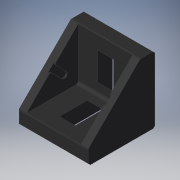
# Autodesk Inventor part: 14073
Saved by Autodesk Inventor 2019 (Build 230136000, 136)
## iProperties
Created: 2023-03-27
Part Number: 14073
Material: Generic
Catalog Web Link: www.cadenas.de
Description: 14071, 14073-2 Hole Inside Corner Brackets
Vendor: 8020
Document SubType Name: Modeling
Designer: psAdmin
Manufacturer: 8020
Mass: 7.49289 g
Surface Area: 51.4239 cm^2
Volume: 7.49289 cm^3
Density: 1 g/cm^3
Appearance: PSOLRGB-175-175-175
Category: PARTsolutions
Company: 8020
Title: 14073
Author: Cadenas PARTsolutions
Comments: 2 Hole Inside Corner Brackets
PSOL_IDENT_0: {$CADENAS_DATA/23d-libs/8020/metric/joining_plates/14071.prj},157 {VTYP=3D},{NB=14073},{LINA=14073},
PSOL_IDENT_1: {NN=14071, 14073},{DATE=31.07.2020 09:21:28},{GEOMDATE=27.02.2012 05:57:00},{VERSION=},{LINEID=10},{
PSOL_IDENT_2: WBVAR=D},{WBNUMERIC=}  {NB=14073},{LINA=14073},{KT=DUMMY},{PN=14073},{MAT=Die-Cast Aluminum},{FIN=Na
PSOL_IDENT_3: tural Finish},{A=27.00},{B=6.40},{C=28.00},{D=8.00},{D1=0.000},{T=3.00},{W=.02},{CC=8-30},{T1=6.000}
PSOL_IDENT_4: ,{CH=0.70710678},{CH1=0.837049},{R=1.000},{A1=5.500},{A2=11.25735931},{A3=17.35400000},{C1=22.000},{
PSOL_IDENT_5: C2=2.82842712},{C3=11.000},{C4=4.94974747},{T2=2.500},{B1=15.34314575},{B2=10.34314575},{B3=5.000},{
PSOL_IDENT_6: D2=0.83704910},{D3=4.24264069},{D4=2.12132034},{E=8.000},{E1=1.400},{E2=3.400}
NB: 14073
NN: 14071, 14073
NT: 2 Hole Inside Corner Brackets
NBSYN: $PN.
LINA: 14073
CATALOG: 80/20
PN: 14073
MAT: Die-Cast Aluminum
FIN: Natural Finish
A: 27
B: 6.4
C: 28
D: 8.00
T: 3
W: .02
CC: 8-30
SUPPLIER: 8020
ARTICLENO: 14073
BOMINFO: 14073
CREATOR: CADENAS GmbH
Autodesk Inventor part; units mm, degrees
ref_plane "YZ Plane" through (0, 0, 0) normal (1, 0, 0) x (0, 1, 0)
ref_plane "XZ Plane" through (0, 0, 0) normal (0, 1, 0) x (-1, 0, 0)
ref_plane "XY Plane" through (0, 0, 0) normal (0, 0, 1) x (1, 0, 0)
sketch "Sketch_1" plane through (0, 0, 0) normal (1, 0, 0) x (0, 1, 0)
  line L0 (5.5858, 27) -> (0.837, 27)
  line L1 (0.837, 27) -> (0, 26.163)
  line L2 (0, 26.163) -> (0, 0.7071)
  line L3 (0, 0.7071) -> (0.7071, 0)
  line L4 (0.7071, 0) -> (26.163, 0)
  line L5 (26.163, 0) -> (27, 0.837)
  line L6 (27, 0.837) -> (27, 5.5858)
  arc A0 (27, 5.5858) -> (26.7071, 6.2929) centre (26, 5.5858) ccw
  line L7 (26.7071, 6.2929) -> (6.2929, 26.7071)
  arc A1 (6.2929, 26.7071) -> (5.5858, 27) centre (5.5858, 26) ccw
  constraints: 16 end point, 4 point on circle, 2 centre point
extrude "Extrusion1" add sketch "Sketch_1" along normal mid plane 28
sketch "Sketch_2" plane through (0, 0, 0) normal (1, 0, 0) x (0, 1, 0)
  line L0 (27, 27) -> (6, 27)
  line L1 (6, 27) -> (6, 7)
  arc A0 (6, 7) -> (7, 6) centre (7, 7) ccw
  line L2 (7, 6) -> (27, 6)
  line L3 (27, 6) -> (27, 27)
  constraints: 8 end point, 2 point on circle, 1 centre point
extrude "Extrusion2" cut sketch "Sketch_2" along normal mid plane 22
sketch "Sketch_3" plane through (0, 0, 0) normal (1, 0, 0) x (0, 1, 0)
  line L0 (6, 21.5) -> (0, 21.5)
  line L1 (0, 21.5) -> (0, 4.146)
  line L2 (0, 4.146) -> (6, 10.2426)
  line L3 (6, 10.2426) -> (6, 21.5)
  constraints: 8 end point
extrude "Extrusion3" cut sketch "Sketch_3" along normal mid plane 6.4
sketch "Sketch_4" plane through (0, 0, 0) normal (1, 0, 0) x (0, 1, 0)
  line L0 (10.2426, 6) -> (4.146, 0)
  line L1 (4.146, 0) -> (21.5, 0)
  line L2 (21.5, 0) -> (21.5, 6)
  line L3 (21.5, 6) -> (10.2426, 6)
  constraints: 8 end point
extrude "Extrusion4" cut sketch "Sketch_4" along normal mid plane 6.4
sketch "Sketch_5" plane through (0, 0, 0) normal (1, 0, 0) x (0, 1, 0)
  line L0 (0, 2.8284) -> (0, 0)
  line L1 (0, 0) -> (2.8284, 0)
  line L2 (2.8284, 0) -> (0, 2.8284)
  constraints: 6 end point
extrude "Extrusion5" cut sketch "Sketch_5" along normal mid plane 22
sketch "Sketch_6" plane through (0, 0, 0) normal (1, 0, 0) x (0, 1, 0)
  line L0 (0, 4.9497) -> (0, 0)
  line L1 (0, 0) -> (4.9497, 0)
  line L2 (4.9497, 0) -> (2.8284, 2.1213)
  line L3 (2.8284, 2.1213) -> (2.1213, 1.4142)
  line L4 (2.1213, 1.4142) -> (1.4142, 2.1213)
  line L5 (1.4142, 2.1213) -> (2.1213, 2.8284)
  line L6 (2.1213, 2.8284) -> (0, 4.9497)
  constraints: 14 end point
extrude "Extrusion6" cut sketch "Sketch_6" along normal mid plane 11
sketch "Sketch_7" plane through (11, 0, 0) normal (1, 0, 0) x (0, 0, -1)
  line L0 (-2.5, 8.1569) -> (0, 5.6569)
  line L1 (0, 5.6569) -> (0, 21)
  line L2 (0, 21) -> (-2.5, 18.5)
  line L3 (-2.5, 18.5) -> (-2.5, 8.1569)
  constraints: 8 end point
extrude "Extrusion7" cut sketch "Sketch_7" against normal blind 5
sketch "Sketch_9" plane through (11, 0, 0) normal (1, 0, 0) x (0, 0, -1)
  line L0 (-21, 0) -> (-5.6569, 0)
  line L1 (-5.6569, 0) -> (-8.1569, 2.5)
  line L2 (-8.1569, 2.5) -> (-18.5, 2.5)
  line L3 (-18.5, 2.5) -> (-21, 0)
  constraints: 8 end point
extrude "Extrusion8" cut sketch "Sketch_9" against normal blind 5
sketch "Sketch_8" plane through (-11, 0, 0) normal (1, 0, 0) x (0, 0, -1)
  line L0 (-2.5, 8.1569) -> (0, 5.6569)
  line L1 (0, 5.6569) -> (0, 21)
  line L2 (0, 21) -> (-2.5, 18.5)
  line L3 (-2.5, 18.5) -> (-2.5, 8.1569)
  constraints: 8 end point
extrude "Extrusion9" cut sketch "Sketch_8" along normal blind 5
sketch "Sketch_10" plane through (-11, 0, 0) normal (1, 0, 0) x (0, 0, -1)
  line L0 (-21, 0) -> (-5.6569, 0)
  line L1 (-5.6569, 0) -> (-8.1569, 2.5)
  line L2 (-8.1569, 2.5) -> (-18.5, 2.5)
  line L3 (-18.5, 2.5) -> (-21, 0)
  constraints: 8 end point
extrude "Extrusion10" cut sketch "Sketch_10" along normal blind 5
sketch "Sketch_11" plane through (0, 0, 0) normal (1, 0, 0) x (0, 1, 0)
  line L0 (0, 26.163) -> (0, 21.9203)
  line L1 (0, 21.9203) -> (2.1213, 24.0416)
  line L2 (2.1213, 24.0416) -> (0, 26.163)
  constraints: 6 end point
extrude "Extrusion11" cut sketch "Sketch_11" along normal mid plane 11
sketch "Sketch_12" plane through (-11, 0, 0) normal (1, 0, 0) x (0, 0, -1)
  arc A0 (-16.6768, 14.909) -> (-18.091, 14.909) centre (-17.3839, 14.2019) ccw
  line L0 (-16.6768, 14.909) -> (-12.6109, 10.8431)
  arc A1 (-12.6109, 10.8431) -> (-10.8431, 10.8431) centre (-11.727, 11.727) ccw
  arc A2 (-10.8431, 10.8431) -> (-10.8431, 12.6109) centre (-11.727, 11.727) ccw
  line L1 (-10.8431, 12.6109) -> (-14.909, 16.6768)
  arc A3 (-14.909, 18.091) -> (-14.909, 16.6768) centre (-14.2019, 17.3839) ccw
  line L2 (-14.909, 18.091) -> (-18.091, 14.909)
  constraints: 8 point on circle, 6 end point, 4 centre point
extrude "Extrusion12" cut sketch "Sketch_12" against normal blind 0.6
sketch "Sketch_13" plane through (11, 0, 0) normal (1, 0, 0) x (0, 0, -1)
  arc A0 (-16.6768, 14.909) -> (-18.091, 14.909) centre (-17.3839, 14.2019) ccw
  line L0 (-16.6768, 14.909) -> (-12.6109, 10.8431)
  arc A1 (-12.6109, 10.8431) -> (-10.8431, 10.8431) centre (-11.727, 11.727) ccw
  arc A2 (-10.8431, 10.8431) -> (-10.8431, 12.6109) centre (-11.727, 11.727) ccw
  line L1 (-10.8431, 12.6109) -> (-14.909, 16.6768)
  arc A3 (-14.909, 18.091) -> (-14.909, 16.6768) centre (-14.2019, 17.3839) ccw
  line L2 (-14.909, 18.091) -> (-18.091, 14.909)
  constraints: 8 point on circle, 6 end point, 4 centre point
extrude "Extrusion13" cut sketch "Sketch_13" along normal blind 0.6
sketch "Sketch_14" plane through (0, 0, 0) normal (1, 0, 0) x (0, 1, 0)
  line L0 (24.0416, 2.1213) -> (21.9203, 0)
  line L1 (21.9203, 0) -> (26.163, 0)
  line L2 (26.163, 0) -> (24.0416, 2.1213)
  constraints: 6 end point
extrude "Extrusion14" cut sketch "Sketch_14" along normal mid plane 11
sketch "Sketch_15" plane through (0, 0, 0) normal (1, 0, 0) x (0, 1, 0)
  line L0 (25.173, 0.9899) -> (22.7688, -1.4142)
  line L1 (22.7688, -1.4142) -> (23.7588, -2.4042)
  line L2 (23.7588, -2.4042) -> (26.163, 0)
  line L3 (26.163, 0) -> (25.173, 0.9899)
  constraints: 8 end point
extrude "Extrusion15" add sketch "Sketch_15" along normal mid plane 8
sketch "Sketch_16" plane through (0, 0, 0) normal (1, 0, 0) x (0, 1, 0)
  line L0 (0, 26.163) -> (-2.4042, 23.7588)
  line L1 (-2.4042, 23.7588) -> (-1.4142, 22.7688)
  line L2 (-1.4142, 22.7688) -> (0.9899, 25.173)
  line L3 (0.9899, 25.173) -> (0, 26.163)
  constraints: 8 end point
extrude "Extrusion16" add sketch "Sketch_16" along normal mid plane 8
sketch "Sketch_17" plane through (0, 0, 0) normal (1, 0, 0) x (0, 1, 0)
  line L0 (3.5355, 1.4142) -> (1.1314, -0.9899)
  line L1 (1.1314, -0.9899) -> (2.1213, -1.9799)
  line L2 (2.1213, -1.9799) -> (4.5255, 0.4243)
  line L3 (4.5255, 0.4243) -> (3.5355, 1.4142)
  constraints: 8 end point
extrude "Extrusion17" add sketch "Sketch_17" along normal mid plane 8
sketch "Sketch_18" plane through (0, 0, 0) normal (1, 0, 0) x (0, 1, 0)
  line L0 (0.4243, 4.5255) -> (-1.9799, 2.1213)
  line L1 (-1.9799, 2.1213) -> (-0.9899, 1.1314)
  line L2 (-0.9899, 1.1314) -> (1.4142, 3.5355)
  line L3 (1.4142, 3.5355) -> (0.4243, 4.5255)
  constraints: 8 end point
extrude "Extrusion18" add sketch "Sketch_18" along normal mid plane 8
body "Solid1"
